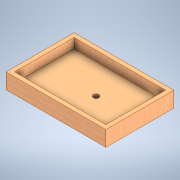
# Autodesk Inventor part: base
Saved by Autodesk Inventor 2020 (Build 240168000, 168)
## iProperties
Created: 2020-05-18
Part Number: base
Material: Wood (Cherry)
Document SubType Name: Modeling
Designer: Manish
Density: 0.63 g/cm^3
Appearance: Cherry - Natural Low Gloss
Author: Manish
Autodesk Inventor part; units mm, degrees
ref_plane "YZ Plane" through (0, 0, 0) normal (1, 0, 0) x (0, 1, 0)
ref_plane "XZ Plane" through (0, 0, 0) normal (0, 1, 0) x (-1, 0, 0)
ref_plane "XY Plane" through (0, 0, 0) normal (0, 0, 1) x (1, 0, 0)
sketch "Sketch3" plane through (0, 0, 0) normal (1, 0, 0) x (0, 1, 0)
  line L0 (0, 0) -> (55, 0)
  line L1 (55, 0) -> (55, -242)
  line L2 (55, -242) -> (0, -242)
  line L3 (0, -242) -> (0, 0)
  dimension "d4" = 55
  dimension "d5" = 242
  constraints: 8 end point, 2 parallel, 1 horizontal, 1 perpendicular
  measures "d4" distance of L1.end L2.end
  measures "d5" distance of L0.end L1.end
extrude "Extrusion3" add sketch "Sketch3" along normal blind 355
sketch "Sketch7" plane through (0, 55, 0) normal (0, 1, 0) x (1, 0, 0)
  circle A0 centre (200, 120) radius 10
  point P0 (0, 0)
  dimension "d20" = 20
  constraints: 1 centre point
  measures "d20" diameter of A0
extrude "Extrusion7" cut sketch "Sketch7" against normal through all
sketch "Sketch8" plane through (0, 55, 0) normal (0, 1, 0) x (1, 0, 0)
  line L0 (15, 15) -> (340, 15)
  line L1 (340, 15) -> (340, 227)
  line L2 (340, 227) -> (15, 227)
  line L3 (15, 227) -> (15, 15)
  line L4 (355, 242) -> (355, 0) projected
  line L5 (0, 242) -> (355, 242) projected
  point P0 (0, 0)
  dimension "d23" = 15
  dimension "d24" = 15
  constraints: 8 end point, 2 parallel, 1 horizontal, 1 perpendicular
  measures "d23" distance between parallel lines of L1 L4
  measures "d24" distance between parallel lines of L2 L5
extrude "Extrusion8" cut sketch "Sketch8" against normal blind 35
body "Solid2"
